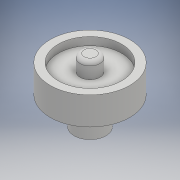
# Autodesk Inventor part: ArmClutchInsert
Saved by Autodesk Inventor 2017 (Build 210142000, 142)
## iProperties
Created: 2017-02-07
Part Number: ArmClutchInsert
Material: Generic
Document SubType Name: Modeling
Designer: aribu
Density: 1 g/cm^3
Appearance: Default
Author: aribu
Autodesk Inventor part; units mm, degrees
ref_plane "YZ Plane" through (0, 0, 0) normal (1, 0, 0) x (0, 1, 0)
ref_plane "XZ Plane" through (0, 0, 0) normal (0, 1, 0) x (-1, 0, 0)
ref_plane "XY Plane" through (0, 0, 0) normal (0, 0, 1) x (1, 0, 0)
sketch "Sketch1" plane through (0, 0, 0) normal (0, 0, 1) x (1, 0, 0)
  circle A0 centre (0, 0) radius 10
  dimension "d0" = 20
  constraints: 1 centre point, 1 coincident
  measures "d0" diameter of A0
extrude "Extrusion1" add sketch "Sketch1" along normal blind 5
sketch "Sketch2" plane through (0, 0, 0) normal (0, 0, -1) x (-1, 0, 0)
  circle A0 centre (0, 0) radius 4
  dimension "d3" = 8
  constraints: 1 centre point, 1 coincident
  measures "d3" diameter of A0
extrude "Extrusion2" add sketch "Sketch2" along normal blind 7
sketch "Sketch3" plane through (0, 0, 5) normal (0, 0, 1) x (1, 0, 0)
  circle A0 centre (0, 0) radius 2.5
  dimension "d6" = 5
  constraints: 1 centre point, 1 coincident
  measures "d6" diameter of A0
extrude "Extrusion3" add sketch "Sketch3" along normal blind 4
fillet "Fillet1" radius 1 1 edges at (-2.5, 0, 9)
sketch "Sketch4" plane through (0, 0, 5) normal (0, 0, 1) x (1, 0, 0)
  circle A0 centre (0, 0) radius 8
  circle A1 centre (0, 0) radius 10
  dimension "d10" = 2
  dimension "d11" = 20
  constraints: 2 centre point, 2 coincident
  measures "d10" radial gap between concentric circles of A1 A0
  measures "d11" diameter of A1
extrude "Extrusion4" add sketch "Sketch4" along normal blind 2
sketch "Sketch5" plane through (0, 0, -7) normal (0, 0, -1) x (-1, 0, 0)
  line L0 (2.5, 1) -> (2.5, -1)
  line L1 (-2.5, -1) -> (-2.5, 1)
  line L2 (-1, 2.5) -> (1, 2.5)
  line L3 (1, -2.5) -> (-1, -2.5)
  line L4 (-2.5, 1) -> (-1, 1)
  line L5 (1, 1) -> (2.5, 1)
  line L6 (-1, -2.5) -> (-1, -1)
  line L7 (-1, 1) -> (-1, 2.5)
  line L8 (2.5, -1) -> (1, -1)
  line L9 (-1, -1) -> (-2.5, -1)
  line L10 (1, 2.5) -> (1, 1)
  line L11 (1, -1) -> (1, -2.5)
  point P0 (0, 0)
  dimension "d14" = 5
  dimension "d15" = 5
  dimension "d16" = 2
  dimension "d17" = 2
  dimension "d20" = 2.5
  dimension "d21" = 2.5
  constraints: 24 end point, 10 parallel, 4 perpendicular, 3 horizontal
  measures "d14" distance of L1.end L0.start
  measures "d15" distance of L3.end L2.start
  measures "d16" distance of L0.start L0.end
  measures "d17" distance of L2.start L2.end
  measures "d20" distance from line of point (0, 0) L0
  measures "d21" distance from line of L2 point (0, 0)
extrude "Extrusion5" cut sketch "Sketch5" against normal blind 10
body "Solid1"
